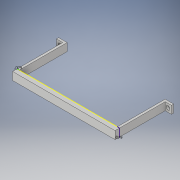
# Autodesk Inventor part: Part1
Saved by Autodesk Inventor 2019 (Build 230136000, 136)
## iProperties
Created: 2020-11-04
Part Number: Part1
Material: Generic
Document SubType Name: Modeling
Designer: johnh
Density: 1 g/cm^3
Appearance: Default
Author: johnh
Autodesk Inventor part; units mm, degrees
ref_plane "YZ Plane" through (0, 0, 0) normal (1, 0, 0) x (0, 1, 0)
ref_plane "XZ Plane" through (0, 0, 0) normal (0, 1, 0) x (-1, 0, 0)
ref_plane "XY Plane" through (0, 0, 0) normal (0, 0, 1) x (1, 0, 0)
sketch "Sketch1" plane through (0, 0, 0) normal (0, 0, 1) x (1, 0, 0)
  line L0 (0, 0) -> (88, 0)
  line L1 (88, 0) -> (88, 7)
  line L2 (88, 7) -> (0, 7)
  line L3 (0, 7) -> (0, 0)
  dimension "d0" = 88
  dimension "d1" = 7
  constraints: 8 end point, 2 parallel, 1 horizontal, 1 perpendicular
  measures "d0" distance of L2.end L1.end
  measures "d1" distance of L2.end L0.start
extrude "Extrusion1" add sketch "Sketch1" along normal blind 4
sketch "Sketch2" plane through (0, 0, 0) normal (0, 0, -1) x (-1, 0, 0)
  line L0 (0, 0) -> (-88, 0) projected
  line L1 (0, 7) -> (0, 0) projected
  line L2 (-88, 7) -> (0, 7) projected
  line L3 (-88, 0) -> (-88, 7) projected
  line L4 (0, 0) -> (2, 0)
  line L5 (2, 0) -> (2, 7)
  line L6 (2, 7) -> (0, 7)
  line L7 (0, 7) -> (0, 0)
  line L8 (-88, 7) -> (-90, 7)
  line L9 (-90, 7) -> (-90, 0)
  line L10 (-90, 0) -> (-88, 0)
  line L11 (-88, 0) -> (-88, 7)
  dimension "d4" = 2
  dimension "d5" = 2
  constraints: 16 end point, 4 parallel, 2 horizontal, 2 perpendicular, 1 point on line
  measures "d4" distance of L6.end L5.end
  measures "d5" distance of L10.end L9.end
extrude "Extrusion2" add sketch "Sketch2" along normal blind 41 contours L1 L6 L5 L4 | L10 L9 L8 L3
extrude "Extrusion3" add sketch "Sketch2" against normal blind 4 contours L1 L6 L5 L4 | L10 L9 L8 L3
sketch "Sketch3" plane through (0, 0, -41) normal (0, 0, -1) x (-1, 0, 0)
  line L0 (-88, 7) -> (-90, 7) projected
  line L1 (-90, 7) -> (-90, 0) projected
  line L2 (-90, 0) -> (-88, 0) projected
  line L3 (-88, 0) -> (-88, 7) projected
  line L4 (2, 0) -> (2, 7) projected
  line L5 (0, 0) -> (2, 0) projected
  line L6 (2, 0) -> (2, 7) projected
  line L7 (2, 7) -> (0, 7) projected
  line L8 (0, 7) -> (0, 0) projected
  line L9 (-88, 0) -> (-95.62, 0)
  line L10 (-95.62, 0) -> (-95.62, 7)
  line L11 (-95.62, 7) -> (-88, 7)
  line L12 (-88, 7) -> (-88, 0)
  circle A0 centre (-92.5085, 3.5) radius 1.75
  line L13 (0, 7) -> (7.62, 7)
  line L14 (7.62, 7) -> (7.62, 0)
  line L15 (7.62, 0) -> (0, 0)
  line L16 (0, 0) -> (0, 7)
  circle A1 centre (4.5085, 3.5) radius 1.75
  dimension "d10" = 3.5
  dimension "d12" = 3.5
  dimension "d17" = 7.62
  dimension "d18" = 7.62
  dimension "d21" = 97.017
  constraints: 16 end point, 4 parallel, 2 centre point, 2 horizontal, 2 perpendicular
  measures "d10" diameter of A0
  measures "d12" diameter of A1
  measures "d17" distance of L2.end L9.end
  measures "d18" distance of L14.end L15.end
  measures "d21" distance of A1.centre A0.centre
extrude "Extrusion4" add sketch "Sketch3" along normal blind 2
body "Solid1"
